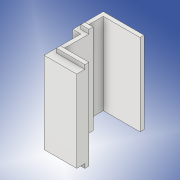
# Autodesk Inventor part: BA003
Saved by Autodesk Inventor 2017 SP1 (Build 210196100, 196)
## iProperties
Created: 2017-06-15
Part Number: BA003
Material: ABS Plastic
Document SubType Name: Modeling
Designer: zallen
Density: 1.06 g/cm^3
Appearance: CR White
Author: zallen
Autodesk Inventor part; units mm, degrees
ref_plane "YZ Plane" through (0, 0, 0) normal (1, 0, 0) x (0, 1, 0)
ref_plane "XZ Plane" through (0, 0, 0) normal (0, 1, 0) x (-1, 0, 0)
ref_plane "XY Plane" through (0, 0, 0) normal (0, 0, 1) x (1, 0, 0)
sketch "Sketch1" plane through (0, 0, 0) normal (0, 0, 1) x (1, 0, 0)
  line L0 (0, 0) -> (40, 0)
  line L1 (40, 0) -> (40, 100)
  line L2 (40, 100) -> (0, 100)
  line L3 (0, 100) -> (0, 0)
  dimension "d0" = 40
  dimension "d1" = 100
  constraints: 8 end point, 2 parallel, 1 horizontal, 1 perpendicular
  measures "d0" distance of L2.end L1.end
  measures "d1" distance of L1.end L0.end
extrude "Extrusion1" add sketch "Sketch1" along normal blind 45
sketch "Sketch2" plane through (0, 0, 0) normal (0, 0, -1) x (-1, 0, 0)
  line L0 (-40, 0) -> (-40, 100) projected
  line L1 (-40, 100) -> (10, 100)
  line L2 (10, 100) -> (10, 0)
  line L3 (10, 0) -> (-40, 0)
  line L4 (-40, 0) -> (-40, 100)
  point P0 (0, 0)
  dimension "d4" = 10
  constraints: 8 end point, 2 parallel, 1 horizontal, 1 horizontal alignment, 1 perpendicular
  measures "d4" distance from line of point (0, 0) L2
extrude "Extrusion2" add sketch "Sketch2" along normal blind 37.5
sketch "Sketch3" plane through (40, 0, 45) normal (1, 0, 0) x (0, 0, -1)
  line L0 (82.5, 100) -> (0, 100) projected
  line L1 (0, 0) -> (0, 100) projected
  line L2 (82.5, 0) -> (0, 0) projected
  line L3 (82.5, 100) -> (82.5, 0) projected
  line L4 (5, 5) -> (5, 95)
  line L5 (5, 95) -> (77.5, 95)
  line L6 (77.5, 95) -> (77.5, 5)
  line L7 (77.5, 5) -> (5, 5)
  point P0 (45, 0)
  dimension "d7" = 5
  constraints: 8 end point, 3 other
  measures "d7" distance between parallel lines of L2 L7
extrude "Extrusion3" cut sketch "Sketch3" against normal blind 35 contours L4 L5 L6 L7
sketch "Sketch4" plane through (5, 0, 45) normal (1, 0, 0) x (0, 0, -1)
  line L0 (45, 100) -> (45, 0) projected
  line L1 (45, 100) -> (82.5, 100) projected
  line L2 (82.5, 0) -> (82.5, 100) projected
  line L3 (45, 0) -> (82.5, 0) projected
  line L4 (50, 5) -> (50, 95)
  line L5 (50, 95) -> (77.5, 95)
  line L6 (77.5, 95) -> (77.5, 5)
  line L7 (77.5, 5) -> (50, 5)
  point P0 (45, 0)
  dimension "d10" = 5
  constraints: 8 end point, 3 other
  measures "d10" distance between parallel lines of L0 L4
extrude "Extrusion4" cut sketch "Sketch4" against normal blind 10 contours L4 L5 L6 L7
sketch "Sketch5" plane through (0, 0, 45) normal (0, -1, 0) x (1, 0, 0)
  line L0 (0, 0) -> (40, 0) projected
  line L1 (0, -45) -> (0, 0) projected
  line L2 (-10, -45) -> (0, -45) projected
  line L3 (-10, -45) -> (-10, -82.5) projected
  line L4 (40, -82.5) -> (-10, -82.5) projected
  line L5 (40, -77.5) -> (-5, -77.5)
  line L6 (-5, -77.5) -> (-5, -50)
  line L7 (-5, -50) -> (5, -50)
  line L8 (5, -50) -> (5, -5)
  line L9 (5, -5) -> (40, -5)
  line L10 (40, -77.5) -> (40, -5)
  line L11 (40, -82.5) -> (40, 0) projected
  dimension "d13" = 5
  constraints: 12 end point, 1 collinear, 4 other
  measures "d13" distance between parallel lines of L4 L5
extrude "Extrusion5" cut sketch "Sketch5" against normal through all contours L10 L5 L6 L7 L8 L9
sketch "Sketch6" plane through (0, 100, 45) normal (0, 1, 0) x (1, 0, 0)
  line L0 (0, 45) -> (0, 0) projected
  line L1 (0, 0) -> (40, 0)
  line L2 (40, 0) -> (40, 10)
  line L3 (40, 10) -> (0, 10)
  line L4 (0, 10) -> (0, 0)
  dimension "d16" = 40
  dimension "d17" = 10
  constraints: 8 end point, 2 parallel, 1 horizontal, 1 perpendicular
  measures "d16" distance of L3.end L2.end
  measures "d17" distance of L2.end L1.end
extrude "Extrusion6" add sketch "Sketch6" against normal blind 100
sketch "Sketch8" plane through (40, 100, 35) normal (0, 0, -1) x (-1, 0, 0)
  line L0 (35, 0) -> (35, -100) projected
  line L1 (0, 0) -> (35, 0) projected
  line L2 (0, 0) -> (0, -100) projected
  line L3 (35, -100) -> (0, -100) projected
  line L4 (35, -105) -> (0, -105)
  line L5 (0, -105) -> (0, 5)
  line L6 (0, 5) -> (35, 5)
  line L7 (35, 5) -> (35, -105)
  point P0 (40, -100)
  dimension "d20" = 5
  dimension "d21" = 5
  constraints: 8 end point, 2 parallel, 1 horizontal, 1 perpendicular, 1 point on line
  measures "d20" distance between parallel lines of L4 L3
  measures "d21" distance between parallel lines of L1 L6
extrude "Extrusion7" add sketch "Sketch8" along normal blind 5
sketch "Sketch10" plane through (5, 0, -5) normal (0, 0, -1) x (-1, 0, 0)
  line L0 (0, 0) -> (0, 100) projected
  line L1 (10, 0) -> (0, 0) projected
  line L2 (10, 0) -> (10, 100) projected
  line L3 (0, 100) -> (10, 100) projected
  line L4 (-35, -5) -> (0, -5) projected
  line L5 (10, 0) -> (0, 0)
  line L6 (0, 0) -> (0, -5)
  line L7 (0, -5) -> (10, -5)
  line L8 (10, -5) -> (10, 0)
  line L9 (0, 105) -> (0, 100) projected
  line L10 (10, 100) -> (0, 100)
  line L11 (0, 100) -> (0, 105)
  line L12 (0, 105) -> (10, 105)
  line L13 (10, 105) -> (10, 100)
  point P0 (5, 0)
  constraints: 16 end point, 4 parallel, 2 horizontal, 2 perpendicular
extrude "Extrusion8" add sketch "Sketch10" along normal blind 5
body "Solid1"
